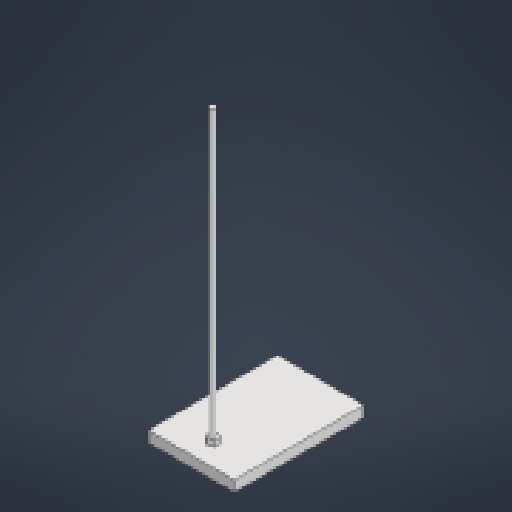
# Autodesk Inventor part: Ring Stand
Saved by Autodesk Inventor 2023.1 (Build 271208000, 208)
## iProperties
Created: 2022-12-06
Part Number: Ring Stand
Material: Generic
Document SubType Name: Modeling
Designer: aubrey-work
Density: 1 g/cm^3
Appearance: Default
Author: aubrey-work
Autodesk Inventor part; units mm, degrees
ref_plane "YZ Plane" through (0, 0, 0) normal (1, 0, 0) x (0, 1, 0)
ref_plane "XZ Plane" through (0, 0, 0) normal (0, 1, 0) x (-1, 0, 0)
ref_plane "XY Plane" through (0, 0, 0) normal (0, 0, 1) x (1, 0, 0)
sketch "Sketch1" plane through (0, 0, 0) normal (0, 1, 0) x (-1, 0, 0)
  line L0 (0, 0) -> (203.2, 0)
  line L1 (203.2, 0) -> (203.2, -304.8)
  line L2 (203.2, -304.8) -> (0, -304.8)
  line L3 (0, -304.8) -> (0, 0)
  dimension "d0" = 203.2
  dimension "d1" = 304.8
  constraints: 8 end point, 2 parallel, 1 horizontal, 1 perpendicular
  measures "d0" distance of L1.end L2.end
  measures "d1" distance of L0.end L1.end
extrude "Extrusion1" add sketch "Sketch1" along normal blind 25.4
sketch "Sketch2" plane through (0, 25.4, 0) normal (0, 1, 0) x (1, 0, 0)
  line L0 (-203.2, 0) -> (0, 0) construction
  line L1 (-101.6, 0) -> (-101.6, 50.8) construction
  line L2 (-101.6, 63.6316) -> (-90.4875, 57.2158)
  line L3 (-90.4875, 57.2158) -> (-90.4875, 44.3842)
  line L4 (-90.4875, 44.3842) -> (-101.6, 37.9684)
  line L5 (-101.6, 37.9684) -> (-112.7125, 44.3842)
  line L6 (-112.7125, 44.3842) -> (-112.7125, 57.2158)
  line L7 (-112.7125, 57.2158) -> (-101.6, 63.6316)
  dimension "d4" = 50.8
  dimension "d9" = 22.225
  constraints: 14 end point, 2 vertical, 1 coincident, 1 midpoint, 13 other
  measures "d4" distance of L1.start L1.end
  measures "d9" distance between parallel lines of L3 L6
extrude "Extrusion2" add sketch "Sketch2" along normal blind 12.3031
sketch "Sketch3" plane through (0, 37.7031, 0) normal (0, 1, 0) x (1, 0, 0)
  line L0 (-112.7125, 57.2158) -> (-112.7125, 44.3842) projected
  line L1 (-112.7125, 44.3842) -> (-101.6, 37.9684) projected
  line L2 (-101.6, 37.9684) -> (-90.4875, 44.3842) projected
  line L3 (-90.4875, 44.3842) -> (-90.4875, 57.2158) projected
  line L4 (-90.4875, 57.2158) -> (-101.6, 63.6316) projected
  line L5 (-101.6, 63.6316) -> (-112.7125, 57.2158) projected
  line L6 (-101.6, 37.9684) -> (-112.7125, 44.3842) construction
  line L7 (-101.6, 63.6316) -> (-101.6, 37.9684) construction
  circle A0 centre (-101.6, 50.8) radius 6.35
  point P0 (0, 0)
  dimension "d8" = 12.7
  constraints: 2 end point, 1 centre point, 1 midpoint, 1 vertical
  measures "d8" diameter of A0
extrude "Extrusion3" add sketch "Sketch3" along normal blind 670.56 contours A0
body "Solid1"
